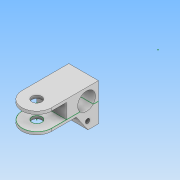
# Autodesk Inventor part: 萬象塊
Saved by Autodesk Inventor 2021 (Build 250183000, 183)
## iProperties
Created: 2025-12-12
Part Number: 萬象塊
Material: 一般
Document SubType Name: Modeling
Designer: User
Density: 1 g/cm^3
Appearance: 預設
Author: User
Autodesk Inventor part; units mm, degrees
ref_plane "YZ Plane" through (0, 0, 0) normal (1, 0, 0) x (0, 1, 0)
ref_plane "XZ Plane" through (0, 0, 0) normal (0, 1, 0) x (-1, 0, 0)
ref_plane "XY Plane" through (0, 0, 0) normal (0, 0, 1) x (1, 0, 0)
sketch "草圖1" plane through (0, 0, 0) normal (1, 0, 0) x (0, 1, 0)
  circle A0 centre (212.2024, 875) radius 90
  line L0 (152.2024, 1000) -> (352.2024, 1000)
  line L1 (352.2024, 1000) -> (352.2024, 785)
  circle A1 centre (32.2024, 865) radius 22.5
  line L2 (-154.9405, 785) -> (152.2024, 1000)
  line L3 (352.2024, 735) -> (352.2024, 1000)
  line L4 (-226.369, 735) -> (352.2024, 735)
  line L5 (152.2024, 1000) -> (-226.369, 735)
  line L6 (123.631, 980) -> (332.2024, 980)
  line L7 (332.2024, 980) -> (332.2024, 755)
  line L8 (332.2024, 755) -> (-47.7976, 755)
  line L9 (-47.7976, 755) -> (-47.7976, 860)
  line L10 (-47.7976, 860) -> (123.631, 980)
  circle A2 centre (212.2024, 875) radius 90
  circle A3 centre (32.2024, 865) radius 22.5
  point P0 (0, 0)
  dimension "d8" = 20
  dimension "d9" = 20
  dimension "d10" = 20
  dimension "d11" = 400
  constraints: 23 end point, 4 centre point, 2 coincident, 2 concentric, 2 parallel, 2 point on line, 1 collinear, 1 horizontal, 1 vertical
  measures "d8" distance between parallel lines of L0 L6
  measures "d9" distance between parallel lines of L1 L7
  measures "d10" distance between parallel lines of L4 L8
  measures "d11" distance between parallel lines of L1 L9
extrude "擠出1" add sketch "草圖1" along normal mid plane 300 contours L6 L7 L8 L9 L2
sketch "草圖2" plane through (-150, 332.2024, 980) normal (0, 1, 0) x (1, 0, 0)
  line L0 (0, 0) -> (300, 0) projected
  line L1 (300, 225) -> (300, 0) projected
  line L2 (300, 225) -> (0, 225) projected
  line L3 (0, 0) -> (0, 225) projected
  circle A0 centre (150, -250) radius 50
  circle A1 centre (150, -250) radius 150
  line L4 (0, 0) -> (300, 0) projected
  line L5 (0, 0) -> (0, -250)
  line L6 (300, 225) -> (300, 0) projected
  line L7 (300, 0) -> (300, -250)
  point P0 (150, 980)
  point P1 (150, 0)
  dimension "d14" = 250
  dimension "d15" = 100
  constraints: 4 end point, 4 tangent, 2 centre point, 2 point on circle, 1 midpoint, 1 vertical alignment
  measures "d14" distance from line of L0 A0.centre
  measures "d15" diameter of A0
extrude "擠出2" add sketch "草圖2" against normal blind 208.571 contours L0 L7 A1 L5 | A1
sketch "草圖3" plane through (150, 0, 0) normal (1, 0, 0) x (0, 0, -1)
  line L0 (-1230, 332.2024) -> (-1230, 332.2024) projected
  line L1 (-1230, 332.2024) -> (-1230, 123.6314) projected
  line L2 (-1230, 123.6314) -> (-1230, 123.6314) projected
  line L3 (-1230, 332.2024) -> (-1230, 123.6314) projected
  line L4 (-755, 332.2024) -> (-1230, 332.2024) projected
  line L5 (-1230, 332.2024) -> (-1230, 123.6314) projected
  line L6 (-980, 123.6314) -> (-1230, 123.6314) projected
  line L7 (-980, 123.6314) -> (-980, 123.631) projected
  line L8 (-980, 123.631) -> (-860, -47.7976) projected
  line L9 (-860, -47.7976) -> (-755, -47.7976) projected
  line L10 (-755, -47.7976) -> (-755, 332.2024) projected
  circle A0 centre (-875, 212.2024) radius 90 projected
  circle A1 centre (-865, 32.2024) radius 22.5 projected
  line L11 (-1380, 302.9169) -> (-1080, 302.9169)
  line L12 (-1080, 302.9169) -> (-1080, 152.9169)
  line L13 (-1080, 152.9169) -> (-1380, 152.9169)
  line L14 (-1380, 152.9169) -> (-1380, 302.9169)
  line L15 (-1380, 332.2024) -> (-1380, 123.6314) projected
  line L16 (-1380, 123.6314) -> (-1230, 123.6314) projected
  line L17 (-1230, 332.2024) -> (-1380, 332.2024) projected
  point P0 (0, 0)
  point P1 (-1380, 227.9169)
  point P2 (-1230, 227.9169)
  dimension "d18" = 150
  dimension "d19" = 300
  constraints: 8 end point, 3 midpoint, 2 parallel, 1 horizontal, 1 horizontal alignment, 1 perpendicular
  measures "d18" distance of L11.end L12.end
  measures "d19" distance of L11.start L11.end
extrude "擠出3" cut sketch "草圖3" against normal through all contours L11 L12 L13 L1 | L1 L13 L14 L11
thread "螺紋1" size "M45x4.5" class "6H" standard "ANSI Metric M Profile" full length
sketch "草圖4" plane through (150, 152.9169, 1230) normal (0, 1, 0) x (1, 0, 0)
  line L0 (0, 150) -> (-300, 150) projected
  line L1 (-300, 0) -> (-300, 150) projected
  arc A0 (-300, 0) -> (0, 0) centre (-150, 0) ccw projected
  line L2 (0, 150) -> (0, 0) projected
  line L3 (0, 287.2857) -> (0, 150) projected
  line L4 (-300, 287.2857) -> (0, 287.2857) projected
  line L5 (-300, 150) -> (-300, 287.2857) projected
  line L6 (-300, 422.7143) -> (-300, 475) projected
  line L7 (-300, 475) -> (0, 475) projected
  line L8 (0, 475) -> (0, 422.7143) projected
  line L9 (0, 422.7143) -> (-300, 422.7143) projected
  circle A1 centre (-150, 0) radius 50 projected
  point P0 (-150, 1230)
